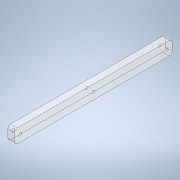
# Autodesk Inventor part: 103.018.01_Distanz_Wand
Saved by Autodesk Inventor 2021 (Build 250183000, 183)
## iProperties
Created: 2021-11-29
Part Number: 103.018.01_Distanz_Wand
Material: Generisch
Document SubType Name: Modeling
Designer: Oliver Ungerer
Density: 1 g/cm^3
Appearance: Wasserblasen
Author: Oliver Ungerer
Autodesk Inventor part; units mm, degrees
ref_plane "YZ Plane" through (0, 0, 0) normal (1, 0, 0) x (0, 1, 0)
ref_plane "XZ Plane" through (0, 0, 0) normal (0, 1, 0) x (-1, 0, 0)
ref_plane "XY Plane" through (0, 0, 0) normal (0, 0, 1) x (1, 0, 0)
sketch "Skizze1" plane through (0, 0, 0) normal (1, 0, 0) x (0, 1, 0)
  line L0 (10, 115) -> (-10, 115)
  line L1 (-10, 115) -> (-10, -115)
  line L2 (-10, -115) -> (10, -115)
  line L3 (10, -115) -> (10, 115)
  line L4 (10, 115) -> (-10, -115) construction
  line L5 (-10, 115) -> (10, -115) construction
  point P0 (0, 0)
  dimension "d0" = 230
  dimension "d1" = 20
  constraints: 12 end point, 2 midpoint, 2 parallel, 1 horizontal, 1 perpendicular
  measures "d0" distance between parallel lines of L2 L0
  measures "d1" distance between parallel lines of L1 L3
extrude "Extrusion1" add sketch "Skizze1" along normal blind 10
sketch "Skizze2" plane through (0, 0, 0) normal (-1, 0, 0) x (0, 0, 1)
  line L0 (-115, -10) -> (-115, 10) projected
  point P0 (0, 0)
  point P1 (-107, 0)
  point P2 (0, 0)
  point P3 (107, 0)
  dimension "d4" = 8
  dimension "d5" = 107
  dimension "d13" = 107
  constraints: 2 horizontal alignment, 1 coincident
  measures "d4" distance from line of L0 point (-107, 0)
  measures "d5" distance of point (0, 0) point (-107, 0)
  measures "d13" distance of point (107, 0) point (0, 0)
hole "Bohrung1" at (0, 0, -107) at (0, 0, 0) at (0, 0, 107) direction (1, 0, 0) diameter 4.5 end through all
fillet "Rundung1" radius 4 4 edges at (5, 10, -115) (5, -10, -115) (5, -10, 115) (5, 10, 115)
